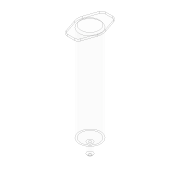
# Autodesk Inventor part: 10 mL syringe
Saved by Autodesk Inventor 2020 (Build 240168000, 168)
## iProperties
Created: 2021-07-28
Part Number: 10 mL syringe
Material: Generic
Document SubType Name: Modeling
Designer: ferrerx
Density: 1 g/cm^3
Appearance: Clear - Light
Mass: 8.54917 g
Surface Area: 81.3891 cm^2
Volume: 8.54917 cm^3
Author: ferrerx
Autodesk Inventor part; units mm, degrees
ref_plane "YZ Plane" through (0, 0, 0) normal (1, 0, 0) x (0, 1, 0)
ref_plane "XZ Plane" through (0, 0, 0) normal (0, 1, 0) x (-1, 0, 0)
ref_plane "XY Plane" through (0, 0, 0) normal (0, 0, 1) x (1, 0, 0)
sketch "Sketch1" plane through (0, 0, 0) normal (0, 1, 0) x (-1, 0, 0)
  circle A0 centre (0, 0) radius 8.35
  circle A1 centre (0, 0) radius 7.1
  dimension "d0" = 16.7
  dimension "d1" = 14.2
  constraints: 2 centre point, 2 coincident
  measures "d0" diameter of A0
  measures "d1" diameter of A1
extrude "Extrusion1" add sketch "Sketch1" along normal blind 75
sketch "Sketch2" plane through (0, 75, 0) normal (0, 1, 0) x (1, 0, 0)
  circle A0 centre (0, 0) radius 9.5
  circle A1 centre (0, 0) radius 7.1
  line L0 (9.5, -15) -> (-9.5, -15) construction
  line L1 (-9.5, -15) -> (-9.5, 15) construction
  line L2 (-9.5, 15) -> (9.5, 15) construction
  line L3 (9.5, 15) -> (9.5, -15) construction
  line L4 (9.5, -15) -> (-9.5, 15) construction
  line L5 (-9.5, -15) -> (9.5, 15) construction
  line L6 (5, 15) -> (-5, 15)
  line L7 (-5, 15) -> (-9.0094, 3.0135)
  line L8 (-9.0094, 3.0135) -> (9, 3.0414) construction
  line L9 (9, 3.0414) -> (5, 15)
  line L10 (0, 0) -> (-9.5, 0) construction
  line L11 (5, -15) -> (-5, -15)
  line L12 (-5, -15) -> (-9.0094, -3.0135)
  line L13 (9, -3.0414) -> (5, -15)
  point P0 (-9.0094, -3.0135)
  dimension "d4" = 14.2
  dimension "d5" = 19
  dimension "d6" = 30
  dimension "d7" = 5
  dimension "d8" = 5
  constraints: 28 end point, 4 symmetric about line, 3 midpoint, 2 centre point, 2 coincident, 2 parallel, 2 point on circle, 2 point on line, 1 horizontal, 1 perpendicular, 1 tangent
  measures "d4" diameter of A1
  measures "d5" diameter of A0
  measures "d6" distance of L0.end L1.end
  measures "d7" horizontal distance of point (0, 0) L6.start
  measures "d8" horizontal distance of point (0, 0) L6.end
extrude "Extrusion2" add sketch "Sketch2" along normal blind 1.5
sketch "Sketch3" plane through (0, 0, 0) normal (0, 0, 1) x (1, 0, 0)
  line L0 (8.35, 0) -> (-8.35, 0) projected
  line L1 (-8.35, 0) -> (-2.3, -2.7)
  line L2 (-2.3, -2.7) -> (0, -2.7)
  line L3 (0, -2.7) -> (0, 0) construction
  line L4 (-8.35, 0) -> (0, 0)
  line L5 (-5, 76.5) -> (5, 76.5) projected
  line L6 (-8.35, 0) -> (0, 0)
  line L7 (0, -2.7) -> (0, 0)
  line L8 (0, -18.54) -> (0, 92.34) projected
  dimension "d11" = 79.2
  dimension "d12" = 2.3
  constraints: 12 end point, 2 collinear, 2 symmetric about line, 1 parallel, 1 point on line, 1 vertical
  measures "d11" distance between parallel lines of L5 L2
  measures "d12" distance of L1.end L2.end
revolve "Revolution1" add sketch "Sketch3" angle 360 about axis through (0, 0, 0) along (0, 1, 0)
sketch "Sketch4" plane through (0, -2.7, 0) normal (0, -1, 0) x (1, 0, 0)
  circle A0 centre (0, 0) radius 2.3
  circle A1 centre (0, 0) radius 1
  circle A2 centre (0, 0) radius 2.3 projected
  dimension "d14" = 2
  constraints: 2 centre point, 2 coincident, 1 concentric
  measures "d14" diameter of A1
extrude "Extrusion3" add sketch "Sketch4" along normal blind 9
chamfer "Chamfer1" distance 1 angle 45 1 edges at (-2.3, -11.7, 0)
fillet "Fillet1" radius 3 4 edges at (5, 75.75, -15) (5, 75.75, 15) (-5, 75.75, -15) (-5, 75.75, 15)
sketch "Sketch5" plane through (0, 75, 0) normal (0, -1, 0) x (1, 0, 0)
  circle A0 centre (0, 0) radius 8.7914
  circle A1 centre (0, 0) radius 2.3 projected
  circle A2 centre (0, 0) radius 8.35
  constraints: 2 centre point, 2 coincident
extrude "Extrusion4" [suppressed]
body "Solid1"
